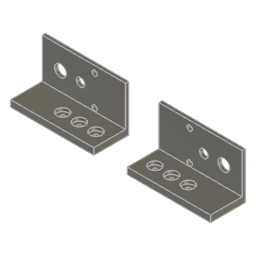
Motor bracket (Autodesk Fusion 360 design; units mm, degrees)
part number: 2026-02-08-23-01-52-319
Autodesk Fusion 360 part; units mm, degrees
sketch "Sketch1" plane through (0, 0, 0) normal (0, 0, 1) x (1, 0, 0)
  line L0 (0, 0) -> (50, 0)
  line L1 (50, 0) -> (50, 22)
  line L2 (50, 22) -> (0, 22)
  line L3 (0, 22) -> (0, 0)
  dimension "d1" = 50
  dimension "d2" = 22
  constraint horizontal L0
  constraint vertical L1
  constraint horizontal L2
  constraint vertical L3
  constraint coincident L0.start L3.end
  measures "d1" distance of L0.start L0.end
  measures "d2" distance of L0.start L2.end
extrude "Extrude1" add sketch "Sketch1" along normal blind 25 makes body 1
sketch "Sketch2" plane through (0, 0, 25) normal (0, 0, 1) x (-1, 0, 0)
  line L0 (0, -22) -> (0, 0)
  line L1 (0, 0) -> (-50, 0)
  line L2 (-50, 0) -> (-50, -22)
  line L3 (-50, -22) -> (0, -22)
  line L4 (-50, 0) -> (0, 0)
  line L5 (0, 0) -> (0, -20)
  line L6 (0, -20) -> (-50, -20)
  line L7 (-50, -20) -> (-50, 0)
  constraint horizontal L4
  constraint vertical L5
  constraint horizontal L6
  constraint vertical L7
  constraint coincident L0 L5.end
  constraint coincident L1.end L2.start
extrude "Extrude2" cut sketch "Sketch2" against normal blind 21 contours L0 L1 L2 L4 L5 L6 L7 bodies 1
sketch "Sketch3" plane through (0, 0, 0) normal (0, 1, 0) x (1, 0, 0)
sketch "Sketch4" plane through (0, 0, 25) normal (0, 0, 1) x (-1, 0, 0)
  line L0 (0, -20) -> (-50, -20)
  line L1 (-50, -20) -> (-50, -22)
  line L2 (-50, -22) -> (0, -22)
  line L3 (0, -22) -> (0, -20)
  line L4 (0, -20) -> (-50, -20)
  line L5 (-50, -20) -> (-50, -22)
  line L6 (-50, -22) -> (0, -22)
  line L7 (0, -22) -> (0, -20)
  constraint horizontal L4
  constraint vertical L5
  constraint horizontal L6
  constraint vertical L7
  constraint coincident L1.end L2.start
  constraint coincident L0.start L3.end
extrude "Extrude3" add sketch "Sketch4" along normal blind 3 bodies 1
sketch "Sketch5" plane through (0, 0, 0) normal (0, 1, 0) x (1, 0, 0)
  circle A0 centre (31.5, -24) radius 1.6
  circle A1 centre (11, -15) radius 3.5
  circle A2 centre (31.5, -5.8915) radius 1.6
  dimension "d11" = 3.2
  dimension "d14" = 7
  dimension "d16" = 3.2
  measures "d11" diameter of A0
  measures "d14" diameter of A1
  measures "d16" diameter of A2
sketch "Sketch6" plane through (0, 0, 0) normal (0, 1, 0) x (1, 0, 0)
  circle A0 centre (23, -15) radius 2.5
  dimension "d18" = 5
  measures "d18" diameter of A0
extrude "Extrude4" cut sketch "Sketch6" sketch "Sketch5" along normal blind 25 of sketch 2 bodies 1
ref_plane "WorkPlane1" through (60, 11, 14) normal (1, 0, 0) x (0, 1, 0)
sketch "Sketch7" plane through (0, 0, 0) normal (0, -1, 0) x (1, 0, 0)
  line L0 (50, 4) -> (0, 4)
  line L1 (0, 4) -> (0, 0)
  line L2 (0, 0) -> (50, 0)
  line L3 (50, 0) -> (50, 4)
sketch "Sketch8" plane through (0, 0, 0) normal (0, 0, 1) x (1, 0, 0)
extrude "Extrude5" cut sketch "Sketch7" against normal blind 1 bodies 1
sketch "Sketch9" plane through (0, 0, 4) normal (0, 0, 1) x (-1, 0, 0)
  line L0 (0, -1) -> (-50, -1)
  line L1 (-50, -1) -> (-50, -20)
  line L2 (-50, -20) -> (0, -20)
  line L3 (0, -20) -> (0, -1)
sketch "Sketch10" plane through (0, 20, 0) normal (0, -1, 0) x (1, 0, 0)
  circle A0 centre (109, 15) radius 3.5
  circle A1 centre (97, 15) radius 2.5
  circle A2 centre (88.5, 5.8915) radius 1.6
  circle A3 centre (88.5, 24) radius 1.6
  line L0 (120, 4) -> (120, 28)
  line L1 (120, 28) -> (70, 28)
  line L2 (70, 28) -> (70, 4)
  line L3 (70, 4) -> (120, 4)
sketch "Sketch11" plane through (0, 0, 4) normal (0, 0, 1) x (-1, 0, 0)
  circle A0 centre (-42.33, -10) radius 1.1
  circle A1 centre (-32.33, -10) radius 1.1
  circle A2 centre (-22.33, -10) radius 1.1
  circle A3 centre (-22.33, -10) radius 3.5
  circle A4 centre (-32.33, -10) radius 3.5
  circle A5 centre (-42.33, -10) radius 3.5
  dimension "d30" = 2.2
  dimension "d31" = 10
  dimension "d32" = 2.2
  dimension "d33" = 10
  dimension "d34" = 2.2
  dimension "d37" = 7
  dimension "d38" = 7
  dimension "d39" = 7
  constraint concentric A2 A3
  constraint concentric A1 A4
  constraint concentric A0 A5
  measures "d30" diameter of A0
  measures "d31" distance of A0.centre A1.centre
  measures "d32" diameter of A1
  measures "d33" distance of A1.centre A2.centre
  measures "d34" diameter of A2
  measures "d37" diameter of A3
  measures "d38" diameter of A4
  measures "d39" diameter of A5
extrude "Extrude6" cut sketch "Sketch11" against normal blind 21 contours A0 | A1 | A2 bodies 1
sketch "Sketch12" plane through (0, 20, 0) normal (0, -1, 0) x (1, 0, 0)
extrude "Extrude7" cut sketch "Sketch11" against normal blind 2 bodies 1
mirror "Mirror2" about plane through (60, 11, 14) normal (1, 0, 0) of bodies 1 makes body 2
